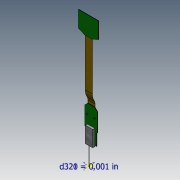
# Autodesk Inventor part: NEUROPIXEL 3A PROBE
Saved by Autodesk Inventor 2018.3 (Build 223284000, 284)
## iProperties
Created: 2017-08-07
Material: Generic
Vendor: IMEC
Document SubType Name: Modeling
Designer: ARNOLDJ
Density: 1 g/cm^3
Appearance: Dark Green
Description: NEUROPIXEL 3A PROBE
RuleStatus: InUse
AfterDocSave0: file://Part Number Cleaner
DESIGN DEPARTMENT: HHMI: JRC - ID&F
ALTERED ITEM PART NUMBER: N/A
ALTERED ITEM VENDOR: N/A
ALTERED ITEM DESCRIPTION: N/A
Author: ARNOLDJ
Revision Number: 0
Autodesk Inventor part; units mm, degrees
sketch "Sketch1" plane through (0, 0, 0) normal (0, 0, 1) x (1, 0, 0)
  line L0 (0, 133.1936) -> (0, -174.4071) projected
  line L1 (-82.221, 0) -> (96.7133, 0) projected
  line L2 (-11.8429, 78.7589) -> (29.9826, 78.7589) construction
  line L3 (29.9826, 78.7589) -> (29.9826, -20.6399) construction
  line L4 (29.9826, -20.6399) -> (-11.8429, -20.6399) construction
  line L5 (-11.8429, -20.6399) -> (-11.8429, 78.7589) construction
  line L6 (-7.642, -75.3683) -> (-7.642, -85.3683)
  line L7 (71.1512, 85.7776) -> (64.977, -130.4641) construction
  line L8 (64.977, -130.4641) -> (-56.659, -126.9911) construction
  line L9 (-56.659, -126.9911) -> (-50.4848, 89.2506) construction
  line L10 (-50.4848, 89.2506) -> (71.1512, 85.7776) construction
  line L11 (-1.9685, 9.271) -> (1.9685, 9.271)
  line L12 (1.9685, 9.271) -> (3.556, 7.6835)
  line L13 (3.556, 7.6835) -> (3.556, -2.413)
  line L14 (3.556, -2.413) -> (3.0619, -2.9071)
  line L15 (3.0619, -2.9071) -> (3.0619, -9.271)
  line L16 (3.0619, -9.271) -> (-3.0619, -9.271)
  line L17 (-3.0619, -9.271) -> (-3.0619, -2.9071)
  line L18 (-3.0619, -2.9071) -> (-3.556, -2.413)
  line L19 (-3.556, -2.413) -> (-3.556, 7.6835)
  line L20 (-3.556, 7.6835) -> (-1.9685, 9.271)
  line L21 (0, 0) -> (0, 10.9448)
  line L22 (1.9431, 43.18) -> (-1.9431, 43.18)
  line L23 (-1.9431, 43.18) -> (-1.9431, 9.271)
  line L24 (-1.9431, 9.271) -> (1.9431, 9.271)
  line L25 (1.9431, 9.271) -> (1.9431, 43.18)
  line L26 (1.9431, 43.18) -> (-1.9431, 9.271) construction
  line L27 (-1.9431, 43.18) -> (1.9431, 9.271) construction
  line L28 (-1.9431, 43.18) -> (-5.6134, 44.704)
  line L29 (-5.6134, 44.704) -> (-5.6134, 53.7718)
  line L30 (-5.6134, 53.7718) -> (5.6134, 53.7718)
  line L31 (5.6134, 53.7718) -> (5.6134, 44.704)
  line L32 (5.6134, 44.704) -> (1.9431, 43.18)
  point P0 (0, 26.2255)
  dimension "d175" = 10
  dimension "d243" = 18.542
  dimension "d244" = 9.271
  dimension "d245" = 7.112
  dimension "d246" = 3.937
  dimension "d247" = 11.684
  dimension "d263" = 33.909
  dimension "d264" = 3.8862
  dimension "d265" = 11.2268
  dimension "d266" = 5.6134
  dimension "d267" = 10.5918
  dimension "d268" = 9.0678
  dimension "d269" = 9.0678
  constraints: 46 end point, 9 perpendicular, 5 point on line, 4 parallel, 2 horizontal, 2 midpoint, 2 vertical, 8 other
  measures "d175" distance of L6.start L6.end
  measures "d243" distance between parallel lines of L16 L11
  measures "d244" distance between parallel lines of L1 L11
  measures "d245" distance between parallel lines of L13 L19
  measures "d246" distance of L11.start L11.end
  measures "d247" distance from line of L13.end L11
  measures "d263" distance of L24.end L22.start
  measures "d264" distance of L22.start L22.end
  measures "d265" distance of L29.end L30.end
  measures "d266" distance between parallel lines of L0 L29
  measures "d267" distance between parallel lines of L30 L22
  measures "d268" distance from line of L28.end L30
  measures "d269" distance of L30.end L31.end
ref_plane "Work Plane4" through (0, 0, 1.524) normal (0, 0, 1) x (1, 0, 0)
extrude "Extrusion4" add sketch "Sketch1" along normal blind 0.2032 contours L11 L12 L13 L1 L0 | L0 L1 L19 L20 L11 | L1 L13 L14 L15 L16 L0 | L0 L16 L17 L18 L19 L1
sketch "Sketch3" plane through (0, 0, 0) normal (1, 0, 0) x (0, 1, 0)
  line L0 (0, 49.0501) -> (0, -26.178) projected
  line L1 (9.271, 0.2032) -> (7.6835, 0.2032) projected
  line L2 (-34.4892, 0) -> (68.482, 0) projected
  line L3 (-32.4978, 1.524) -> (56.5338, 1.524) projected
  arc A0 (16.411, 1.524) -> (12.4911, 0.5057) centre (16.411, -6.5303) ccw
  line L4 (16.411, 1.524) -> (43.815, 1.524)
  line L5 (9.271, 0) -> (10.6931, 0)
  arc A1 (10.6931, 0) -> (12.4911, 0.5057) centre (10.5317, 4.0226) ccw
  line L6 (9.271, -0.0227) -> (10.6936, -0.0227)
  arc A2 (10.6936, -0.0227) -> (12.5021, 0.4859) centre (10.5317, 4.0226) ccw
  arc A3 (16.411, 1.5013) -> (12.5021, 0.4859) centre (16.411, -6.5303) ccw
  line L7 (16.411, 1.5013) -> (43.815, 1.5013)
  line L8 (43.815, 1.524) -> (43.815, 1.5013)
  line L9 (9.271, -0.0227) -> (9.271, 0)
  point P0 (0, 0)
  dimension "d301" = 43.815
  constraints: 12 end point, 8 point on circle, 4 centre point, 2 point on line, 2 tangent, 1 horizontal, 1 perpendicular, 1 vertical, 2 other
  measures "d301" distance from line of L4.end L0
ref_plane "Work Plane1" through (0, 0, 0.1778) normal (0, 0, 1) x (1, 0, 0)
sketch "Sketch4" plane through (0, 0, 0.1778) normal (0, 0, 1) x (1, 0, 0)
  point P0 (0, 0)
ref_plane "Work Plane2" through (0, 0, 0.75) normal (0, 0, 1) x (1, 0, 0)
sketch "Sketch10" plane through (0, 0, 1.524) normal (0, 0, 1) x (1, 0, 0)
  line L0 (-5.6134, 53.7718) -> (5.6134, 53.7718) projected
  line L1 (-5.6134, 44.704) -> (-5.6134, 53.7718) projected
  line L2 (5.6134, 53.7718) -> (5.6134, 44.704) projected
  line L3 (5.6134, 44.704) -> (1.9431, 43.18) projected
  line L4 (-1.9431, 43.18) -> (-5.6134, 44.704) projected
  line L5 (-5.6134, 44.704) -> (-5.6134, 53.7718)
  line L6 (-5.6134, 53.7718) -> (5.6134, 53.7718)
  line L7 (5.6134, 53.7718) -> (5.6134, 44.704)
  line L8 (-5.6134, 44.704) -> (-1.9431, 43.18)
  line L9 (5.6134, 44.704) -> (1.9431, 43.18)
  line L10 (1.9431, 43.18) -> (-1.9431, 43.18)
  point P0 (0, 0)
  dimension "d307" = 112.549
  dimension "d308" = 10.5918
  constraints: 12 end point, 4 collinear, 1 horizontal
  measures "d307" angle of L4 L1
  measures "d308" distance between parallel lines of L10 L0
extrude "Extrusion11" add sketch "Sketch10" along normal blind 0.2032
sketch "Sketch9" plane through (0, 0, 0.75) normal (0, 0, 1) x (1, 0, 0)
  point P0 (0, 0)
sketch "Sketch6" plane through (0, 0, 0.2032) normal (0, 0, 1) x (1, 0, 0)
  line L0 (0, 13.081) -> (0, -13.589) projected
  line L1 (-4.9784, 0) -> (4.9784, 0) projected
  line L2 (2.0955, -0.889) -> (-2.0955, -0.889)
  line L3 (-2.0955, -0.889) -> (-2.0955, -9.779)
  line L4 (-2.0955, -9.779) -> (2.0955, -9.779)
  line L5 (2.0955, -9.779) -> (2.0955, -0.889)
  line L6 (2.0955, -0.889) -> (-2.0955, -9.779) construction
  line L7 (-2.0955, -0.889) -> (2.0955, -9.779) construction
  line L8 (-3.0619, -9.271) -> (3.0619, -9.271) projected
  point P0 (0, 0)
  point P1 (0, -5.334)
  dimension "d283" = 4.191
  dimension "d284" = 0.508
  dimension "d285" = 8.89
  constraints: 12 end point, 2 midpoint, 2 parallel, 1 horizontal, 1 perpendicular, 1 point on line
  measures "d283" distance of L3.end L4.end
  measures "d284" distance between parallel lines of L8 L4
  measures "d285" distance of L2.end L3.end
extrude "Extrusion8" add sketch "Sketch6" along normal blind 1.2192
sketch "Sketch7" plane through (-2.0955, -9.779, 0.2032) normal (0, -1, 0) x (1, 0, 0)
  line L0 (0, 0) -> (4.191, 0) projected
  line L1 (4.191, 0) -> (4.191, 1.2192) projected
  line L2 (0, 1.2192) -> (4.191, 1.2192) projected
  line L3 (0, 0) -> (0, 1.2192) projected
  line L4 (2.0955, 1.8694) -> (2.0955, -0.5486) projected
  line L5 (2.1305, 1.1492) -> (2.0605, 1.1492)
  line L6 (2.0605, 1.1492) -> (2.0605, 1.2192)
  line L7 (2.0605, 1.2192) -> (2.1305, 1.2192)
  line L8 (2.1305, 1.2192) -> (2.1305, 1.1492)
  line L9 (2.1305, 1.1492) -> (2.0605, 1.2192) construction
  line L10 (2.0605, 1.1492) -> (2.1305, 1.2192) construction
  point P0 (2.0955, -0.2032)
  point P1 (2.0955, 1.1842)
  dimension "d288" = 0.07
  dimension "d289" = 0.07
  constraints: 12 end point, 2 midpoint, 2 parallel, 2 point on line, 1 horizontal, 1 perpendicular
  measures "d288" distance of L5.end L6.end
  measures "d289" distance of L5.start L5.end
extrude "Extrusion9" add sketch "Sketch7" along normal blind 10 contours L5 L6 L2 L4 | L4 L2 L8 L5
sketch "Sketch8" plane through (0, 0, 0.2032) normal (0, 0, 1) x (1, 0, 0)
  line L0 (2.0955, -0.889) -> (2.0955, -9.271) projected
  line L1 (2.0955, -9.271) -> (3.0619, -9.271) projected
  line L2 (3.0619, -9.271) -> (3.0619, -2.9071) projected
  line L3 (3.0619, -2.9071) -> (3.556, -2.413) projected
  line L4 (3.556, -2.413) -> (3.556, 7.6835) projected
  line L5 (3.556, 7.6835) -> (1.9685, 9.271) projected
  line L6 (1.9685, 9.271) -> (-1.9685, 9.271) projected
  line L7 (-1.9685, 9.271) -> (-3.556, 7.6835) projected
  line L8 (-3.556, 7.6835) -> (-3.556, -2.413) projected
  line L9 (-3.556, -2.413) -> (-3.0619, -2.9071) projected
  line L10 (-3.0619, -2.9071) -> (-3.0619, -9.271) projected
  line L11 (-3.0619, -9.271) -> (-2.0955, -9.271) projected
  line L12 (-2.0955, -9.271) -> (-2.0955, -0.889) projected
  line L13 (-2.0955, -0.889) -> (2.0955, -0.889) projected
  circle A0 centre (-2.14, 4.191) radius 0.4191
  circle A1 centre (2.14, 4.191) radius 0.4191
  point P0 (0, 0)
  dimension "d292" = 4.2799
  dimension "d294" = 2.1399
  dimension "d295" = 0.8382
  dimension "d314" = 5.08
  constraints: 2 centre point, 1 equal radius, 1 horizontal alignment
  measures "d292" distance of A1.centre A0.centre
  measures "d294" horizontal distance of point (0, 0) A0.centre
  measures "d295" diameter of A1
  measures "d314" distance from line of A0.centre L6
extrude "Extrusion10" add sketch "Sketch8" along normal blind 0.508 contours A0 | A1
extrude "Extrusion12" add sketch "Sketch3" along normal mid plane 4.0005 contours L3 L8 L7 A3 A2 L2 A1 A0 | L2 A2 L6 L9
sketch "Sketch11" plane through (-2.0955, -19.779, 0.2032) normal (0, -1, 0) x (1, 0, 0)
  line L0 (2.0605, 1.2192) -> (2.0605, 1.1492) projected
  line L1 (2.0605, 1.1492) -> (2.1305, 1.1492) projected
  line L2 (2.1305, 1.1492) -> (2.1305, 1.2192) projected
  line L3 (2.1305, 1.2192) -> (2.0605, 1.2192) projected
  point P0 (2.0955, -0.2032)
  point P1 (2.0955, 1.1842)
  dimension "d320" = 0.035
  dimension "d321" = 0.035
  measures "d320" distance from line of L2 point (2.095, 1.184)
  measures "d321" distance from line of point (2.095, 1.184) L3
body "Solid2"
